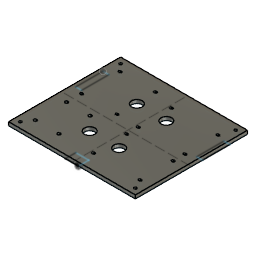
LY1 (Autodesk Fusion 360 design; units mm, degrees)
part number: 2026-02-10-12-12-57-400
part number: 2026-02-10-12-27-31-314
Autodesk Fusion 360 part; units mm, degrees
sketch "Sketch1" plane through (0, 0, 0) normal (0, 0, 1) x (1, 0, 0) in component "Front"
  line L0 (0, 0) -> (230, 0)
  line L1 (230, 0) -> (230, 200)
  line L2 (230, 200) -> (0, 200)
  line L3 (0, 200) -> (0, 0)
  dimension "d3" = 200
  dimension "d4" = 230
  constraint horizontal L0
  constraint vertical L1
  constraint horizontal L2
  constraint vertical L3
  constraint coincident L0.start L3.end
  measures "d3" distance of L0.end L1.end
  measures "d4" distance of L1.end L2.end
sketch "Sketch2" plane through (0, 0, 0) normal (0, 0, 1) x (1, 0, 0) in component "Front"
  line L0 (0, 0) -> (215, 0)
  line L1 (215, 0) -> (215, 190)
  line L2 (215, 190) -> (0, 190)
  line L3 (0, 190) -> (0, 0)
  dimension "d20" = 215
  dimension "d21" = 190
  constraint horizontal L0
  constraint vertical L1
  constraint horizontal L2
  constraint vertical L3
  constraint coincident L0.start L3.end
  measures "d20" distance of L1.end L2.end
  measures "d21" distance of L0.end L1.end
extrude "Extrude1" add sketch "Sketch2" along normal blind 6 in component "Front"
sketch "Sketch3" plane through (0, 0, 6) normal (0, 0, 1) x (-1, 0, 0) in component "Front"
  line L0 (0, -190) -> (0, 0)
  line L1 (0, 0) -> (-215, 0)
  line L2 (-215, 0) -> (-215, -190)
  line L3 (-215, -190) -> (0, -190)
  line L4 (0, -190) -> (0, 0)
  line L5 (-20, -25) -> (-60, -25) construction
  line L6 (-20, -25) -> (-20, -78) construction
  line L7 (-107.5, -190) -> (-107.5, 0) construction
  line L8 (-20, -78) -> (-20, -103) construction
  line L9 (-20, -103) -> (-20, -168) construction
  line L10 (-20, -103) -> (-80, -103) construction
  line L11 (-20.0087, -169.75) -> (-22.195, -169.7391)
  line L12 (-20, -166.25) -> (-22, -166.25)
  line L13 (-80, -169.75) -> (-82, -169.75)
  line L14 (-80, -166.25) -> (-82.1073, -166.25)
  line L15 (-20, -104.75) -> (-22, -104.75)
  line L16 (-20, -101.25) -> (-22, -101.25)
  line L17 (-80, -104.75) -> (-82, -104.75)
  line L18 (-80, -101.25) -> (-82, -101.25)
  arc A0 (-82, -101.25) -> (-82, -104.75) centre (-82, -103) ccw
  arc A1 (-80, -104.75) -> (-80, -101.25) centre (-80, -103) ccw
  arc A2 (-20, -104.75) -> (-20, -101.25) centre (-20, -103) ccw
  arc A3 (-22, -101.25) -> (-22, -104.75) centre (-22, -103) ccw
  arc A4 (-20.0087, -169.75) -> (-20, -166.25) centre (-20, -168) ccw
  arc A5 (-22, -166.25) -> (-21.8223, -169.741) centre (-22, -168) ccw
  line L19 (-20, -168) -> (-20.25, -168) construction
  line L20 (-21.75, -168) -> (-80, -168) construction
  arc A6 (-80, -169.75) -> (-80, -166.25) centre (-80, -168) ccw
  arc A7 (-82, -166.25) -> (-82, -169.75) centre (-82, -168) ccw
  line L21 (-20, -80.2241) -> (-21, -80.2241)
  line L22 (-20, -75.7241) -> (-21.2396, -75.7241)
  arc A8 (-20, -80.2241) -> (-20, -75.7241) centre (-20, -77.9741) ccw
  arc A9 (-21, -75.7241) -> (-21, -80.2241) centre (-21, -77.9741) ccw
  line L23 (-60, -22.75) -> (-61, -22.75)
  line L24 (-60, -27.25) -> (-61, -27.25)
  line L25 (-60, -75.7241) -> (-61, -75.7241)
  line L26 (-60, -80.2241) -> (-61, -80.2241)
  arc A10 (-61, -75.7241) -> (-61, -80.2241) centre (-61, -77.9741) ccw
  arc A11 (-60, -80.2241) -> (-60, -75.7241) centre (-60, -77.9741) ccw
  arc A12 (-60, -27.25) -> (-60, -22.75) centre (-60, -25) ccw
  arc A13 (-60, -27.25) -> (-60, -22.75) centre (-60, -25) ccw
  arc A14 (-60, -27.25) -> (-60, -22.75) centre (-60, -25) ccw
  arc A15 (-61, -22.75) -> (-61, -27.25) centre (-61, -25) ccw
  arc A16 (-20, -27.25) -> (-20.0023, -22.75) centre (-20, -25) ccw
  arc A17 (-20, -27.25) -> (-20.0023, -22.75) centre (-20, -25) ccw
  line L27 (-20, -27.25) -> (-21, -27.25)
  line L28 (-19.9977, -22.75) -> (-21, -22.75)
  arc A18 (-21, -22.75) -> (-21, -27.25) centre (-21, -25) ccw
  arc A19 (-20, -27.25) -> (-19.9977, -22.75) centre (-20, -25) ccw
  arc A20 (-119, -156.25) -> (-119, -159.75) centre (-119, -158) ccw
  line L29 (-117, -159.75) -> (-119, -159.75)
  arc A21 (-117, -159.75) -> (-117, -156.25) centre (-117, -158) ccw
  line L30 (-117, -156.25) -> (-119.1073, -156.25)
  line L31 (-119, -158) -> (-198, -158) construction
  arc A22 (-198, -156.25) -> (-198, -159.75) centre (-198, -158) ccw
  line L32 (-196, -156.25) -> (-198.1073, -156.25)
  line L33 (-196, -159.75) -> (-198, -159.75)
  arc A23 (-196, -159.75) -> (-196, -156.25) centre (-196, -158) ccw
  line L34 (-119, -158) -> (-119, -102) construction
  line L35 (-117, -100.25) -> (-119.1073, -100.25)
  arc A24 (-117, -103.75) -> (-117, -100.25) centre (-117, -102) ccw
  line L36 (-117, -103.75) -> (-119, -103.75)
  arc A25 (-119, -100.25) -> (-119, -103.75) centre (-119, -102) ccw
  arc A26 (-196, -103.75) -> (-196, -100.25) centre (-196, -102) ccw
  line L37 (-196, -100.25) -> (-198.1073, -100.25)
  arc A27 (-198, -100.25) -> (-198, -103.75) centre (-198, -102) ccw
  line L38 (-196, -103.75) -> (-198, -103.75)
  line L39 (-196, -24.25) -> (-198.1073, -24.25)
  line L40 (-119, -82) -> (-198, -82) construction
  arc A28 (-117, -27.75) -> (-117, -24.25) centre (-117, -26) ccw
  line L41 (-119, -82) -> (-119, -26) construction
  line L42 (-196, -80.25) -> (-198.1073, -80.25)
  arc A29 (-119, -80.25) -> (-119, -83.75) centre (-119, -82) ccw
  line L43 (-117, -27.75) -> (-119, -27.75)
  arc A30 (-119, -24.25) -> (-119, -27.75) centre (-119, -26) ccw
  line L44 (-196, -83.75) -> (-198, -83.75)
  line L45 (-117, -24.25) -> (-119.1073, -24.25)
  line L46 (-196, -27.75) -> (-198, -27.75)
  arc A31 (-196, -83.75) -> (-196, -80.25) centre (-196, -82) ccw
  arc A32 (-198, -24.25) -> (-198, -27.75) centre (-198, -26) ccw
  arc A33 (-198, -80.25) -> (-198, -83.75) centre (-198, -82) ccw
  arc A34 (-196, -27.75) -> (-196, -24.25) centre (-196, -26) ccw
  line L47 (-117, -83.75) -> (-119, -83.75)
  arc A35 (-117, -83.75) -> (-117, -80.25) centre (-117, -82) ccw
  line L48 (-117, -80.25) -> (-119.1073, -80.25)
  line L49 (-107.5, -95) -> (0, -95) construction
  circle A36 centre (-10, -180) radius 2.25
  circle A37 centre (-10, -10) radius 2.25
  circle A38 centre (-205, -180) radius 2.25
  circle A39 centre (-205, -10) radius 2.25
  line L50 (-107.5, -95) -> (-132.5, -95) construction
  line L51 (-132.5, -95) -> (-132.5, -135) construction
  line L52 (-132.5, -95) -> (-215, -95) construction
  circle A40 centre (-132.5, -135) radius 9
  circle A41 centre (-132.5, -55) radius 9
  circle A42 centre (-82.5, -135) radius 9
  circle A43 centre (-82.5, -55) radius 9
  line L53 (-82.5, -135) -> (-132.5, -135) construction
  dimension "d26" = 4.5
  dimension "d27" = 40
  dimension "d29" = 53
  dimension "d31" = 4.5
  dimension "d34" = 4.5
  dimension "d36" = 25
  dimension "d37" = 3.5
  dimension "d38" = 65
  dimension "d39" = 3.5
  dimension "d40" = 60
  dimension "d41" = 3.5
  dimension "d42" = 60
  dimension "d44" = 3.5
  dimension "d45" = 3.5
  dimension "d46" = 3.5
  dimension "d47" = 3.5
  dimension "d51" = 4.5
  dimension "d52" = 215
  dimension "d56" = 3.5
  dimension "d57" = 79
  dimension "d60" = 3.5
  dimension "d61" = 56
  dimension "d62" = 3.5
  dimension "d63" = 3.5
  dimension "d64" = 3.5
  dimension "d65" = 79
  dimension "d66" = 3.5
  dimension "d67" = 56
  dimension "d68" = 3.5
  dimension "d69" = 3.5
  dimension "d74" = 4.5
  dimension "d75" = 25
  dimension "d76" = 190
  dimension "d77" = 40
  dimension "d78" = 18
  dimension "d79" = 50
  constraint coincident L0.start L3.end
  constraint coincident L0.end L1.start
  constraint coincident L5.start L6.start
  constraint horizontal L5
  constraint coincident L5.end A12.centre
  constraint perpendicular L5 L6
  constraint midpoint L3 L7.start
  constraint midpoint L1 L7.end
  constraint parallel L6 L8
  constraint coincident L8.end L9.start
  constraint parallel L8 L9
  constraint coincident L9.end A4.centre
  constraint perpendicular L8 L10
  constraint coincident L10.end A1.centre
  constraint perpendicular L9 L19
  constraint coincident L20.end A6.centre
  constraint coincident L11.end A5
  constraint tangent L11 A4
  constraint coincident L9 L12.start
  constraint tangent L12 A5
  constraint perpendicular L9 L12
  constraint tangent L13 A7
  constraint parallel L13 L20
  constraint tangent L14 A6
  constraint parallel L13 L14
  constraint coincident L9 L15.start
  constraint tangent L15 A3
  constraint perpendicular L9 L15
  constraint coincident L8 L16.start
  constraint tangent L16 A3
  constraint tangent L17 A0
  constraint parallel L10 L17
  constraint tangent L18 A0
  constraint parallel L17 L18
  constraint collinear L19 L20
  constraint coincident L11 A5.end
  constraint coincident L14 A7.start
  constraint coincident L8 L21.start
  constraint tangent L21 A9
  constraint perpendicular L8 L21
  constraint coincident L6 L22.start
  constraint tangent L22 A8
  constraint perpendicular L6 L22
  constraint coincident L22 A9.start
  constraint coincident L6 A16.start
  constraint tangent L23 A15
  constraint parallel L5 L23
  constraint parallel L23 L24
  constraint tangent L25 A10
  constraint parallel L24 L25
  constraint tangent L26 A10
  constraint parallel L25 L26
  constraint tangent L27 A18
  constraint horizontal L27
  constraint tangent L28 A18
  constraint coincident L28 A16.end
  constraint tangent A20 L29
  constraint tangent A21 L30
  constraint parallel L29 L30
  constraint coincident A20.start L30
  constraint coincident A20.centre L31.start
  constraint horizontal L31
  constraint tangent A22 L33
  constraint tangent L32 A23
  constraint parallel L32 L33
  constraint coincident A22.start L32
  constraint perpendicular L30 L34
  constraint tangent L36 A25
  constraint tangent L35 A24
  constraint parallel L35 L36
  constraint coincident A25.start L35
  constraint tangent A27 L38
  constraint tangent A26 L37
  constraint parallel L37 L38
  constraint coincident A27.start L37
  constraint tangent A29 L47
  constraint tangent A35 L48
  constraint parallel L47 L48
  constraint coincident A29.start L48
  constraint coincident L40.start L41.start
  constraint horizontal L40
  constraint tangent L44 A33
  constraint tangent L42 A31
  constraint parallel L42 L44
  constraint coincident A33.start L42
  constraint perpendicular L41 L48
  constraint tangent L43 A30
  constraint tangent A28 L45
  constraint parallel L43 L45
  constraint coincident A30.start L45
  constraint tangent L46 A32
  constraint tangent L39 A34
  constraint parallel L39 L46
  constraint coincident A32.start L39
  constraint midpoint L7 L49.start
  constraint midpoint L4 L49.end
  constraint symmetric L49 A36 A37
  constraint symmetric L7 A36 A38
  constraint symmetric L7 A37 A39
  constraint perpendicular L7 L50
  constraint perpendicular L50 L51
  constraint midpoint L2 L52.end
  constraint coincident L51.end A40.centre
  constraint symmetric L52 A40 A41
  constraint symmetric L7 A40 A42
  constraint symmetric L7 A41 A43
  constraint coincident A42.centre L53.start
  measures "d26" diameter of A16
  measures "d27" distance of L5.start L5.end
  measures "d29" distance of L5.start L6.end
  measures "d31" diameter of A12
  measures "d34" diameter of A8
  measures "d36" distance of L6.end L8.end
  measures "d37" diameter of A2
  measures "d38" distance of L8.end L9.end
  measures "d39" diameter of A4
  measures "d40" distance of L8.end L10.end
  measures "d41" diameter of A1
  measures "d42" distance of L9.end L20.end
  measures "d44" diameter of A3
  measures "d45" diameter of A5
  measures "d46" diameter of A0
  measures "d47" diameter of A7
  measures "d51" diameter of A10
  measures "d52" distance of L0.start L2.end
  measures "d56" diameter of A20
  measures "d57" distance of A20.centre L31.end
  measures "d60" diameter of A22
  measures "d61" distance of A20.centre L34.end
  measures "d62" diameter of A25
  measures "d63" diameter of A27
  measures "d64" diameter of A29
  measures "d65" distance of L40.start L40.end
  measures "d66" diameter of A33
  measures "d67" distance of L41.end L40.start
  measures "d68" diameter of A30
  measures "d69" diameter of A32
  measures "d74" diameter of A36
  measures "d75" distance of L49.start L50.end
  measures "d76" distance of L1.end L2.end
  measures "d77" distance of L50.end L51.end
  measures "d78" diameter of A40
  measures "d79" distance of A42.centre L51.end
extrude "Extrude2" cut sketch "Sketch3" against normal blind 7 contours L11 L12 A4 A5 | L11 A5 | L13 L14 A6 A7 | L15 L16 A2 A3 | L17 L18 A0 A1 | L21 L22 A8 A9 | L23 L24 A12 A13 A14 A15 | L25 L26 A10 A11 | A16 A17 L27 L28 A18 A19 | A20 L29 A21 L30 | A22 L32 L33 A23 | L35 A24 L36 A25 | A26 L37 A27 L38 | L39 L46 A32 A34 | A28 L43 A30 L45 | L42 L44 A31 A33 | A29 L47 A35 L48 | A36 | A37 | A38 | A39 | A40 | A41 | A42 | A43 in component "Front"
sketch "Sketch4" plane through (0, 0, 0) normal (0, 0, -1) x (1, 0, 0) in component "Front"
  line L0 (117, -24.25) -> (119, -24.25)
  arc A0 (119, -27.75) -> (119, -24.25) centre (119, -26) ccw
  line L1 (119, -27.75) -> (117, -27.75)
  arc A1 (117, -24.25) -> (117, -27.75) centre (117, -26) ccw
  circle A2 centre (132.5, -135) radius 9
  line L2 (60, -75.7241) -> (61, -75.7241)
  arc A3 (61, -80.2241) -> (61, -75.7241) centre (61, -77.9741) ccw
  line L3 (61, -80.2241) -> (60, -80.2241)
  arc A4 (60, -75.7241) -> (60, -80.2241) centre (60, -77.9741) ccw
  line L4 (117, -100.25) -> (119, -100.25)
  arc A5 (119, -103.75) -> (119, -100.25) centre (119, -102) ccw
  line L5 (119, -103.75) -> (117, -103.75)
  arc A6 (117, -100.25) -> (117, -103.75) centre (117, -102) ccw
  line L6 (20, -101.25) -> (22, -101.25)
  arc A7 (22, -104.75) -> (22, -101.25) centre (22, -103) ccw
  line L7 (22, -104.75) -> (20, -104.75)
  arc A8 (20, -101.25) -> (20, -104.75) centre (20, -103) ccw
  line L8 (20, -166.25) -> (22, -166.25)
  arc A9 (21.8223, -169.741) -> (22, -166.25) centre (22, -168) ccw
  line L9 (21.8223, -169.741) -> (20.0087, -169.75)
  arc A10 (20, -166.25) -> (20.0087, -169.75) centre (20, -168) ccw
  line L10 (80, -166.25) -> (82, -166.25)
  arc A11 (82, -169.75) -> (82, -166.25) centre (82, -168) ccw
  line L11 (82, -169.75) -> (80, -169.75)
  arc A12 (80, -166.25) -> (80, -169.75) centre (80, -168) ccw
  circle A13 centre (205, -180) radius 2.25
  arc A14 (198, -103.75) -> (198, -100.25) centre (198, -102) ccw
  line L12 (198, -103.75) -> (196, -103.75)
  arc A15 (196, -100.25) -> (196, -103.75) centre (196, -102) ccw
  line L13 (196, -100.25) -> (198, -100.25)
  line L14 (20, -75.7241) -> (21, -75.7241)
  arc A16 (21, -80.2241) -> (21, -75.7241) centre (21, -77.9741) ccw
  line L15 (21, -80.2241) -> (20, -80.2241)
  arc A17 (20, -75.7241) -> (20, -80.2241) centre (20, -77.9741) ccw
  circle A18 centre (10, -10) radius 2.25
  line L16 (196, -24.25) -> (198, -24.25)
  arc A19 (198, -27.75) -> (198, -24.25) centre (198, -26) ccw
  line L17 (198, -27.75) -> (196, -27.75)
  arc A20 (196, -24.25) -> (196, -27.75) centre (196, -26) ccw
  line L18 (60, -22.75) -> (61, -22.75)
  arc A21 (61, -27.25) -> (61, -22.75) centre (61, -25) ccw
  line L19 (61, -27.25) -> (60, -27.25)
  arc A22 (60, -22.75) -> (60, -27.25) centre (60, -25) ccw
  circle A23 centre (132.5, -55) radius 9
  line L20 (117, -80.25) -> (119, -80.25)
  arc A24 (119, -83.75) -> (119, -80.25) centre (119, -82) ccw
  line L21 (119, -83.75) -> (117, -83.75)
  arc A25 (117, -80.25) -> (117, -83.75) centre (117, -82) ccw
  line L22 (117, -156.25) -> (119, -156.25)
  arc A26 (119, -159.75) -> (119, -156.25) centre (119, -158) ccw
  line L23 (119, -159.75) -> (117, -159.75)
  arc A27 (117, -156.25) -> (117, -159.75) centre (117, -158) ccw
  line L24 (80, -101.25) -> (82, -101.25)
  arc A28 (82, -104.75) -> (82, -101.25) centre (82, -103) ccw
  line L25 (82, -104.75) -> (80, -104.75)
  arc A29 (80, -101.25) -> (80, -104.75) centre (80, -103) ccw
  circle A30 centre (10, -180) radius 2.25
  circle A31 centre (82.5, -135) radius 9
  line L26 (196, -156.25) -> (198, -156.25)
  arc A32 (198, -159.75) -> (198, -156.25) centre (198, -158) ccw
  line L27 (198, -159.75) -> (196, -159.75)
  arc A33 (196, -156.25) -> (196, -159.75) centre (196, -158) ccw
  line L28 (196, -80.25) -> (198, -80.25)
  arc A34 (198, -83.75) -> (198, -80.25) centre (198, -82) ccw
  line L29 (198, -83.75) -> (196, -83.75)
  arc A35 (196, -80.25) -> (196, -83.75) centre (196, -82) ccw
  circle A36 centre (82.5, -55) radius 9
  line L30 (19.9977, -22.75) -> (21, -22.75)
  arc A37 (21, -27.25) -> (21, -22.75) centre (21, -25) ccw
  line L31 (21, -27.25) -> (20, -27.25)
  arc A38 (19.9977, -22.75) -> (20, -27.25) centre (20, -25) ccw
  circle A39 centre (205, -10) radius 2.25
  line L32 (0, 0) -> (0, -190)
  line L33 (0, -190) -> (215, -190)
  line L34 (215, -190) -> (215, 0)
  line L35 (215, 0) -> (0, 0)
hole "Hole1" at (10, 10, 0) at (205, 10, 0) at (205, 180, 0) at (10, 180, 0) direction (0, 0, 1) diameter 8.4 depth 3 tip angle 150 in component "Front"
sketch "Sketch5" plane through (0, 0, 0) normal (0, 0, -1) x (1, 0, 0) in component "Front"
  circle A0 centre (205, -180) radius 4.2
  circle A1 centre (10, -10) radius 4.2
  circle A2 centre (205, -10) radius 4.2
  circle A3 centre (10, -180) radius 4.2
  line L0 (117, -24.25) -> (119, -24.25)
  arc A4 (119, -27.75) -> (119, -24.25) centre (119, -26) ccw
  line L1 (119, -27.75) -> (117, -27.75)
  arc A5 (117, -24.25) -> (117, -27.75) centre (117, -26) ccw
  circle A6 centre (132.5, -135) radius 9
  line L2 (60, -75.7241) -> (61, -75.7241)
  arc A7 (61, -80.2241) -> (61, -75.7241) centre (61, -77.9741) ccw
  line L3 (61, -80.2241) -> (60, -80.2241)
  arc A8 (60, -75.7241) -> (60, -80.2241) centre (60, -77.9741) ccw
  line L4 (117, -100.25) -> (119, -100.25)
  arc A9 (119, -103.75) -> (119, -100.25) centre (119, -102) ccw
  line L5 (119, -103.75) -> (117, -103.75)
  arc A10 (117, -100.25) -> (117, -103.75) centre (117, -102) ccw
  line L6 (20, -101.25) -> (22, -101.25)
  arc A11 (22, -104.75) -> (22, -101.25) centre (22, -103) ccw
  line L7 (22, -104.75) -> (20, -104.75)
  arc A12 (20, -101.25) -> (20, -104.75) centre (20, -103) ccw
  line L8 (20, -166.25) -> (22, -166.25)
  arc A13 (21.8223, -169.741) -> (22, -166.25) centre (22, -168) ccw
  line L9 (21.8223, -169.741) -> (20.0087, -169.75)
  arc A14 (20, -166.25) -> (20.0087, -169.75) centre (20, -168) ccw
  line L10 (80, -166.25) -> (82, -166.25)
  arc A15 (82, -169.75) -> (82, -166.25) centre (82, -168) ccw
  line L11 (82, -169.75) -> (80, -169.75)
  arc A16 (80, -166.25) -> (80, -169.75) centre (80, -168) ccw
  arc A17 (198, -103.75) -> (198, -100.25) centre (198, -102) ccw
  line L12 (198, -103.75) -> (196, -103.75)
  arc A18 (196, -100.25) -> (196, -103.75) centre (196, -102) ccw
  line L13 (196, -100.25) -> (198, -100.25)
  line L14 (20, -75.7241) -> (21, -75.7241)
  arc A19 (21, -80.2241) -> (21, -75.7241) centre (21, -77.9741) ccw
  line L15 (21, -80.2241) -> (20, -80.2241)
  arc A20 (20, -75.7241) -> (20, -80.2241) centre (20, -77.9741) ccw
  line L16 (196, -24.25) -> (198, -24.25)
  arc A21 (198, -27.75) -> (198, -24.25) centre (198, -26) ccw
  line L17 (198, -27.75) -> (196, -27.75)
  arc A22 (196, -24.25) -> (196, -27.75) centre (196, -26) ccw
  line L18 (60, -22.75) -> (61, -22.75)
  arc A23 (61, -27.25) -> (61, -22.75) centre (61, -25) ccw
  line L19 (61, -27.25) -> (60, -27.25)
  arc A24 (60, -22.75) -> (60, -27.25) centre (60, -25) ccw
  circle A25 centre (132.5, -55) radius 9
  line L20 (117, -80.25) -> (119, -80.25)
  arc A26 (119, -83.75) -> (119, -80.25) centre (119, -82) ccw
  line L21 (119, -83.75) -> (117, -83.75)
  arc A27 (117, -80.25) -> (117, -83.75) centre (117, -82) ccw
  line L22 (117, -156.25) -> (119, -156.25)
  arc A28 (119, -159.75) -> (119, -156.25) centre (119, -158) ccw
  line L23 (119, -159.75) -> (117, -159.75)
  arc A29 (117, -156.25) -> (117, -159.75) centre (117, -158) ccw
  line L24 (80, -101.25) -> (82, -101.25)
  arc A30 (82, -104.75) -> (82, -101.25) centre (82, -103) ccw
  line L25 (82, -104.75) -> (80, -104.75)
  arc A31 (80, -101.25) -> (80, -104.75) centre (80, -103) ccw
  circle A32 centre (82.5, -135) radius 9
  line L26 (196, -156.25) -> (198, -156.25)
  arc A33 (198, -159.75) -> (198, -156.25) centre (198, -158) ccw
  line L27 (198, -159.75) -> (196, -159.75)
  arc A34 (196, -156.25) -> (196, -159.75) centre (196, -158) ccw
  line L28 (196, -80.25) -> (198, -80.25)
  arc A35 (198, -83.75) -> (198, -80.25) centre (198, -82) ccw
  line L29 (198, -83.75) -> (196, -83.75)
  arc A36 (196, -80.25) -> (196, -83.75) centre (196, -82) ccw
  circle A37 centre (82.5, -55) radius 9
  line L30 (19.9977, -22.75) -> (21, -22.75)
  arc A38 (21, -27.25) -> (21, -22.75) centre (21, -25) ccw
  line L31 (21, -27.25) -> (20, -27.25)
  arc A39 (19.9977, -22.75) -> (20, -27.25) centre (20, -25) ccw
  line L32 (0, 0) -> (0, -190)
  line L33 (0, -190) -> (215, -190)
  line L34 (215, -190) -> (215, 0)
  line L35 (215, 0) -> (0, 0)
  line L36 (0, -160) -> (10, -160)
  line L37 (10, -160) -> (10, -114)
  line L38 (10, -114) -> (0, -114)
  line L39 (0, -114) -> (0, -160)
  line L40 (107.5, -190) -> (107.5, 0) construction
  line L41 (0, -95) -> (215, -95) construction
  line L42 (205, -160) -> (205, -114)
  line L43 (205, -114) -> (215, -114)
  line L44 (215, -114) -> (215, -160)
  line L45 (215, -160) -> (205, -160)
  line L46 (107.5, 0) -> (118.5, 0) construction
  line L47 (107.5, 0) -> (96.5, 0) construction
  line L48 (96.5, 0) -> (118.5, 0)
  line L49 (118.5, 0) -> (118.5, -17.4665)
  line L50 (118.5, -17.4665) -> (96.5, -17.4665)
  line L51 (96.5, -17.4665) -> (96.5, 0)
  dimension "d85" = 10
  dimension "d86" = 46
  dimension "d87" = 11
  dimension "d88" = 11
  constraint horizontal L36
  constraint vertical L37
  constraint horizontal L38
  constraint vertical L39
  constraint coincident L32 L36.start
  constraint midpoint L33 L40.start
  constraint midpoint L35 L40.end
  constraint midpoint L32 L41.start
  constraint midpoint L34 L41.end
  constraint symmetric L36.start L40 L44.end
  constraint symmetric L36.end L40 L42.start
  constraint symmetric L37.end L40 L42.end
  constraint symmetric L38.end L40 L43.end
  constraint perpendicular L40 L46
  constraint perpendicular L40 L47
  constraint horizontal L48
  constraint vertical L49
  constraint horizontal L50
  constraint vertical L51
  measures "d85" distance of L37.end L38.end
  measures "d86" distance of L36.start L38.end
  measures "d87" distance of L40.end L46.end
  measures "d88" distance of L40.end L47.end
extrude "Extrude3" [suppressed] in component "Front"
component "Front" placed x (1, 0, 0) y (0, 1, 0) z (0, 0, 1) at (0, 0, 0)
equation "base_thick = 5 mm" comment "base thickeness"
equation "d_small_hole = 3.5 mm" comment "holes for board"
equation "d_medium_hole = 4.5 mm" comment "hole for pillar"
equation "d_big_holes = 18 mm" comment "holes for big cables"
equation "d_motor_external_hole = 7 mm" comment "external where you attach the motors"
equation "b_motore_ext = 46 mm" comment "base of the moto, or external diameter for soppert"
equation "b_motore_int = 38 mm" comment "base of the moto, or internal diameter for soppert"
equation "distance_center_motor = 9.5 mm" comment "distance from the end of motor supprt and the start of th eholes for motor"
equation "side_square = 22 mm" comment "support for bearing"
equation "d_minus_bearing = 6 mm"
equation "d_medium_bearing = 12 mm"
equation "d_bearing = 19 mm"
equation "d_pillar = 8.4 mm"
equation "Length = 215 mm"
equation "Height = 190 mm"
equation "d20 = Length"
equation "d21 = Height"
equation "d26 = d_medium_hole"
equation "d31 = d_medium_hole"
equation "d34 = d_medium_hole"
equation "d37 = d_small_hole"
equation "d39 = d_small_hole"
equation "d41 = d_small_hole"
equation "d44 = d_small_hole"
equation "d45 = d_small_hole"
equation "d46 = d_small_hole"
equation "d47 = d_small_hole"
equation "d51 = d_medium_hole"
equation "d56 = d_small_hole"
equation "d60 = d_small_hole"
equation "d62 = d_small_hole"
equation "d63 = d_small_hole"
equation "d64 = d_small_hole"
equation "d66 = d_small_hole"
equation "d68 = d_small_hole"
equation "d69 = d_small_hole"
equation "d74 = d_medium_hole"
equation "d78 = d_big_holes"
equation "d83 = d_pillar"
